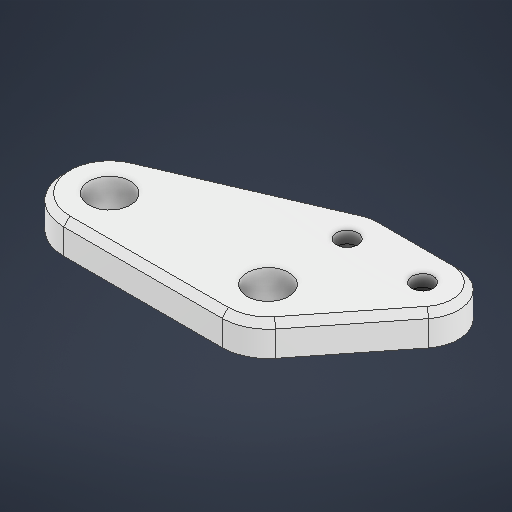
# Autodesk Inventor part: CNC-010-XAxisLimitSwitchMount
Saved by Autodesk Inventor 2026.2 (Build 302298000, 298)
## iProperties
Created: 2026-06-17
Part Number: CNC-010-XAxisLimitSwitchMount
Material: ABS Plastic
Document SubType Name: Modeling
Designer: Kenji
Density: 1.06 g/cm^3
Appearance: Smooth - White
Author: Kenji
Autodesk Inventor part; units mm, degrees
ref_plane "YZ Plane" through (0, 0, 0) normal (1, 0, 0) x (0, 1, 0)
ref_plane "XZ Plane" through (0, 0, 0) normal (0, 1, 0) x (-1, 0, 0)
ref_plane "XY Plane" through (0, 0, 0) normal (0, 0, 1) x (1, 0, 0)
sketch "Sketch1" plane through (0, 0, 0) normal (0, 1, 0) x (-1, 0, 0)
  circle A0 centre (0, 0) radius 2.63
  line L0 (0, 0) -> (0, -2.63) construction
  line L1 (0, 0) -> (2.63, 0) construction
  circle A1 centre (20, 0) radius 2.63
  circle A2 centre (0, -10) radius 1.35
  circle A3 centre (-9.525, -10) radius 1.35
  circle A4 centre (20, 0) radius 5.805 construction
  circle A5 centre (0, 0) radius 5.805 construction
  circle A6 centre (0, -10) radius 4.525 construction
  circle A7 centre (-9.525, -10) radius 4.525 construction
  line L2 (-4.5564, 3.5969) -> (-13.0767, -7.1962)
  line L3 (22.2946, -5.3322) -> (1.7886, -14.1565)
  line L4 (20, 5.805) -> (0, 5.805)
  line L5 (0, -14.525) -> (-9.525, -14.525)
  arc A8 (22.2946, -5.3322) -> (20, 5.805) centre (20, 0) ccw
  arc A9 (0, 5.805) -> (-4.5564, 3.5969) centre (0, 0) ccw
  arc A10 (0, -14.525) -> (1.7886, -14.1565) centre (0, -10) ccw
  arc A11 (-13.0767, -7.1962) -> (-9.525, -14.525) centre (-9.525, -10) ccw
  point P0 (-13.5097, -12.8558)
  dimension "d0" = 5.26
  dimension "d1" = 20
  dimension "d2" = 2.7
  dimension "d3" = 10
  dimension "d4" = 9.525
  dimension "d5" = 3.175
  dimension "d6" = 3.175
  constraints: 18 point on circle, 12 centre point, 12 end point, 8 equal radius, 7 tangent, 2 coincident, 2 point on line, 1 horizontal, 1 horizontal alignment, 1 perpendicular, 1 vertical
  measures "d0" diameter of A0
  measures "d1" distance of point (0, 0) A1.centre
  measures "d2" diameter of A2
  measures "d3" distance of point (0, 0) A2.centre
  measures "d4" distance of A3.centre A2.centre
  measures "d5" radial gap between concentric circles of A4 A1
  measures "d6" radial gap between concentric circles of A6 A2
extrude "Extrusion1" add sketch "Sketch1" along normal blind 4
sketch "Sketch2" plane through (0, 0, 0) normal (0, -1, 0) x (1, 0, 0)
  line L0 (-20, 5.805) -> (0, 5.805) projected
  arc A0 (-20, 5.805) -> (-22.2946, -5.3322) centre (-20, 0) ccw projected
  line L1 (-1.7886, -14.1565) -> (-22.2946, -5.3322) projected
  arc A1 (-1.7886, -14.1565) -> (0, -14.525) centre (0, -10) ccw projected
  line L2 (9.525, -14.525) -> (0, -14.525) projected
  arc A2 (9.525, -14.525) -> (13.0767, -7.1962) centre (9.525, -10) ccw projected
  line L3 (4.5564, 3.5969) -> (13.0767, -7.1962) projected
  arc A3 (4.5564, 3.5969) -> (0, 5.805) centre (0, 0) ccw projected
  circle A4 centre (-20, 0) radius 2.63 projected
  circle A5 centre (9.525, -10) radius 1.35 projected
  circle A6 centre (0, -10) radius 1.35 projected
  circle A7 centre (0, 0) radius 2.63 projected
  circle A8 centre (9.525, -10) radius 2
  circle A9 centre (0, -10) radius 2
  dimension "d9" = 4
  constraints: 2 centre point, 2 coincident, 1 equal radius
  measures "d9" diameter of A8
extrude "Extrusion2" cut sketch "Sketch2" against normal blind 2.5 contours A8 | A9
chamfer "Chamfer1" distance 0.7937 angle 45 8 edges at (-10, 4, 5.805) (2.5316, 4, 5.2239) (8.8165, 4, -1.7997) (13.597, 4, -11.9734) (4.7625, 4, -14.525) (-0.9131, 4, -14.4319) (-12.0416, 4, -9.7444) (-25.6856, 4, 1.1714)
body "Solid1"
